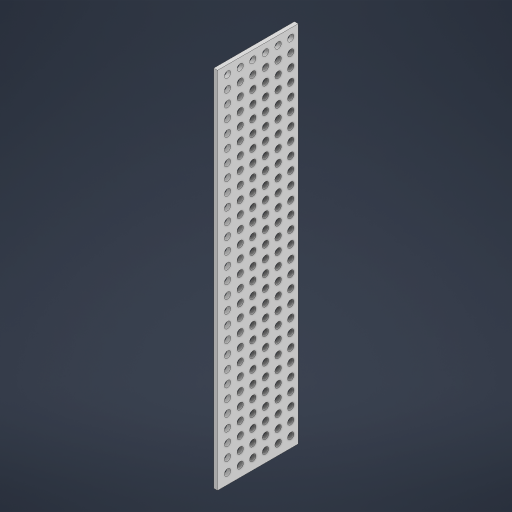
# Autodesk Inventor part: platte_drawing
Saved by Autodesk Inventor 2023 (Build 270158000, 158)
## iProperties
Created: 2022-11-14
Part Number: platte_drawing
Material: Generic
Document SubType Name: Modeling
Designer: bananenbrot
Density: 1 g/cm^3
Appearance: Default
Author: bananenbrot
Autodesk Inventor part; units mm, degrees
ref_plane "YZ Plane" through (0, 0, 0) normal (1, 0, 0) x (0, 1, 0)
ref_plane "XZ Plane" through (0, 0, 0) normal (0, 1, 0) x (-1, 0, 0)
ref_plane "XY Plane" through (0, 0, 0) normal (0, 0, 1) x (1, 0, 0)
sketch "Sketch1" plane through (0, 0, 0) normal (1, 0, 0) x (0, 1, 0)
  line L0 (116.0424, 78.2136) -> (-171.9576, 78.2136)
  line L1 (-171.9576, 78.2136) -> (-171.9576, 14.3136)
  line L2 (-171.9576, 14.3136) -> (116.0424, 14.3136)
  line L3 (116.0424, 14.3136) -> (116.0424, 78.2136)
  point P0 (0, 0)
  dimension "d0" = 63.9
  dimension "d1" = 288
  constraints: 8 end point, 2 parallel, 1 horizontal, 1 perpendicular
  measures "d0" distance of L2.end L0.start
  measures "d1" distance of L0.start L0.end
extrude "Extrusion1" add sketch "Sketch1" along normal blind 3
sketch "Sketch2" plane through (3, 0, 0) normal (1, 0, 0) x (0, 0, -1)
  line L0 (-14.3136, -171.9576) -> (-14.3136, 116.0424) projected
  line L1 (-14.3136, 116.0424) -> (-78.2136, 116.0424) projected
  circle A0 centre (-20.282, 109.2057) radius 2.5
  point P0 (0, 0)
  dimension "d4" = 5
  constraints: 1 centre point
  measures "d4" diameter of A0
extrude "Extrusion2" cut sketch "Sketch2" against normal blind 3
pattern_linear "Rectangular Pattern1" count 28 spacing 10.1 along (0, -1, 0) count 6 spacing 10 along (0, 0, 1) of "Extrusion2"
body "Solid1"
